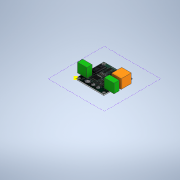
# Autodesk Inventor part: motorcontroller
Saved by Autodesk Inventor 2021.5 (Build 255421000, 421)
## iProperties
Created: 2025-01-01
Part Number: motorcontroller
Material: Generic
Document SubType Name: Modeling
Designer: email
Density: 1 g/cm^3
Appearance: Default
Author: email
Autodesk Inventor part; units mm, degrees
ref_plane "YZ Plane" through (0, 0, 0) normal (1, 0, 0) x (0, 1, 0)
ref_plane "XZ Plane" through (0, 0, 0) normal (0, 1, 0) x (-1, 0, 0)
ref_plane "XY Plane" through (0, 0, 0) normal (0, 0, 1) x (1, 0, 0)
sketch "Sketch1" plane through (0, 0, 0) normal (0, 1, 0) x (-1, 0, 0)
  line L0 (0, 0) -> (-55, 0)
  line L1 (-55, 0) -> (-55, -55)
  line L2 (-55, -55) -> (0, -55)
  line L3 (0, -55) -> (0, 0)
  circle A0 centre (-3.5, -51.5) radius 1.5
  circle A1 centre (-51.5, -51.5) radius 1.5
  circle A2 centre (-3.5, -3.5) radius 1.75
  circle A3 centre (-51.5, -3.5) radius 1.75
  line L4 (-80.9711, 26.8887) -> (29.0289, 26.8887) construction
  line L5 (29.0289, 26.8887) -> (29.0289, -83.1113) construction
  line L6 (29.0289, -83.1113) -> (-80.9711, -83.1113) construction
  line L7 (-80.9711, -83.1113) -> (-80.9711, 26.8887) construction
  dimension "d1" = 55
  dimension "d4" = 55
  dimension "d49" = 3.5
  dimension "d50" = 3.5
  dimension "d51" = 3
  dimension "d54" = 3
  dimension "d55" = 3.5
  dimension "d56" = 3.5
  dimension "d59" = 3.5
  dimension "d60" = 3.5
  dimension "d61" = 3.5
  dimension "d62" = 3.5
  dimension "d63" = 3.5
  dimension "d64" = 3.5
  dimension "d90" = 110
  constraints: 8 end point, 4 centre point, 2 parallel, 1 horizontal, 1 perpendicular, 2 other
  measures "d1" distance of L0.end L1.end
  measures "d4" distance of L1.end L2.end
  measures "d49" distance from line of L2 A0.centre
  measures "d50" distance from line of L3 A0.centre
  measures "d51" diameter of A0
  measures "d54" diameter of A1
  measures "d55" distance from line of L2 A1.centre
  measures "d56" distance from line of L1 A1.centre
  measures "d59" diameter of A2
  measures "d60" diameter of A3
  measures "d61" distance from line of L0 A2.centre
  measures "d62" distance from line of L3 A2.centre
  measures "d63" distance from line of L1 A3.centre
  measures "d64" distance from line of L0 A3.centre
  measures "d90" distance of L6.end L4.start
extrude "Extrusion1" add sketch "Sketch1" along normal blind 2
sketch "Sketch4" plane through (0, 2, 0) normal (0, 1, 0) x (1, 0, 0)
  line L0 (-26.0558, 81.8781) -> (83.9442, 81.8781) construction
  line L1 (83.9442, 81.8781) -> (83.9442, -28.1219) construction
  line L2 (83.9442, -28.1219) -> (-26.0558, -28.1219) construction
  line L3 (-26.0558, -28.1219) -> (-26.0558, 81.8781) construction
  point P0 (0, 0)
  dimension "d77" = 110
  constraints: 2 other
  measures "d77" distance of L0.end L1.end
sketch "Sketch5" plane through (0, 2, 0) normal (0, 1, 0) x (1, 0, 0)
  line L0 (44.5715, 45.2054) -> (63.4108, 45.2054)
  line L1 (63.4108, 45.2054) -> (63.4108, 25.2259)
  line L2 (63.4108, 25.2259) -> (44.5715, 25.2259)
  line L3 (44.5715, 25.2259) -> (44.5715, 45.2054)
  line L4 (45, 21) -> (64, 21)
  line L5 (64, 21) -> (64, 10.8389)
  line L6 (64, 10.8389) -> (45, 10.8389)
  line L7 (45, 10.8389) -> (45, 21)
  line L8 (-7.4993, 21) -> (11, 21)
  line L9 (11, 21) -> (11, 10.8389)
  line L10 (11, 10.8389) -> (-7.4993, 10.8389)
  line L11 (-7.4993, 10.8389) -> (-7.4993, 21)
  point P0 (0, 0)
  constraints: 24 end point, 6 parallel, 3 horizontal, 3 perpendicular
extrude "Extrusion2" add sketch "Sketch5" along normal blind 18
body "Solid1"
